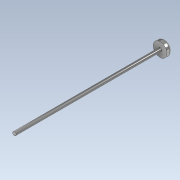
# Autodesk Inventor part: Screw
Saved by Autodesk Inventor 2021 (Build 250183000, 183)
## iProperties
Created: 2021-08-28
Part Number: Screw
Material: Iron, Gray
Document SubType Name: Modeling
Designer: digge
Density: 7.15 g/cm^3
Appearance: Honed
Author: digge
Autodesk Inventor part; units mm, degrees
ref_plane "YZ Plane" through (0, 0, 0) normal (1, 0, 0) x (0, 1, 0)
ref_plane "XZ Plane" through (0, 0, 0) normal (0, 1, 0) x (-1, 0, 0)
ref_plane "XY Plane" through (0, 0, 0) normal (0, 0, 1) x (1, 0, 0)
sketch "Sketch1" plane through (0, 0, 0) normal (0, 1, 0) x (-1, 0, 0)
  line L0 (170, 300) -> (170, 180)
  line L1 (170, 180) -> (174.1898, 180)
  line L2 (174.1898, 180) -> (174.1898, 175.5572)
  line L3 (168.5, 300) -> (168.5, 175.5572)
  line L4 (168.5, 175.5572) -> (174.1898, 175.5572)
  line L5 (170, 300) -> (168.5, 300)
  point P0 (0, 0)
  dimension "d2" = 1.5
  dimension "d3" = 120
  constraints: 12 end point, 3 perpendicular, 1 horizontal, 1 vertical
  measures "d2" distance of L0.start L3.start
  measures "d3" distance between parallel lines of L1 L5
revolve "Revolution1" add sketch "Sketch1" angle 360 about axis through (-168.5, 0, 300) along (0, 0, -1)
fillet "Fillet1" radius 2 1 edges at (-162.8102, 0, 175.5572)
thread "Thread1" size "M3x0.5" class "6g" standard "ANSI Metric M Profile" full length
equation "\"d2\" = 0.5 * ScrewDiameter"
equation "\"d3\" = ScrewLength"
equation "\"ScrewLength\" = 120"
equation "\"ScrewDiameter\" = 3"
body "Solid1"
